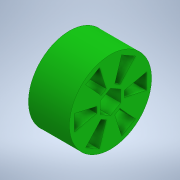
# Autodesk Inventor part: Compliance wheel
Saved by Autodesk Inventor 2021.1 (Build 251245000, 245)
## iProperties
Created: 2020-01-14
Part Number: Compliance wheel
Material: ABS Plastic
Document SubType Name: Modeling
Designer: woodn
Density: 1.06 g/cm^3
Appearance: Dark Green
Author: woodn
Autodesk Inventor part; units mm, degrees
ref_plane "YZ Plane" through (0, 0, 0) normal (1, 0, 0) x (0, 1, 0)
ref_plane "XZ Plane" through (0, 0, 0) normal (0, 1, 0) x (-1, 0, 0)
ref_plane "XY Plane" through (0, 0, 0) normal (0, 0, 1) x (1, 0, 0)
sketch "Sketch1" plane through (0, 0, 0) normal (1, 0, 0) x (0, 1, 0)
  circle A0 centre (0, 0) radius 25.4
  dimension "d16" = 50.8
  constraints: 1 centre point, 1 coincident
  measures "d16" diameter of A0
extrude "Extrusion1" add sketch "Sketch1" along normal blind 25.4
sketch "Sketch2" plane through (25.4, 0, 0) normal (1, 0, 0) x (0, 0, -1)
  circle A0 centre (0, 0) radius 50.8
  circle A1 centre (0, 0) radius 25.4
  line L0 (6.35, 3.6662) -> (6.35, -3.6662)
  line L1 (6.35, -3.6662) -> (0, -7.3323)
  line L2 (0, -7.3323) -> (-6.35, -3.6662)
  line L3 (-6.35, -3.6662) -> (-6.35, 3.6662)
  line L4 (-6.35, 3.6662) -> (0, 7.3323)
  line L5 (0, 7.3323) -> (6.35, 3.6662)
  circle A2 centre (0, 0) radius 44.45
  line L6 (0, 0) -> (-5.6587, 24.7616)
  circle A3 centre (0, 0) radius 25.4 projected
  line L7 (0, 0) -> (5.2266, 24.8564)
  arc A4 (9.1466, 43.4988) -> (-9.9027, 43.3329) centre (0, 0) ccw
  point P0 (5.2266, 24.8564)
  point P1 (-5.6587, 24.7616)
  dimension "d3" = 25.4
  dimension "d4" = 6.35
  dimension "d5" = 0
  dimension "d8" = 6.35
  dimension "d9" = 19.05
  dimension "d10" = 0
  constraints: 16 end point, 6 point on circle, 4 centre point, 2 coincident, 2 point on line, 14 other
  measures "d3" radial gap between concentric circles of A0 A1
  measures "d4" distance from line of point (0, 0) L5
  measures "d5" horizontal distance of point (0, 0) L4.end
  measures "d8" radial gap between concentric circles of A0 A2
  measures "d9" distance of A2.start A2.end
  measures "d10" distance of point (0, 0) A4.centre
extrude "Extrusion4" cut sketch "Sketch2" against normal through all contours L7 L6 L4 L5 | L5 L0 L1 L2 L3 L4 L6 L7
sketch "Sketch3" plane through (25.4, 0, 0) normal (1, 0, 0) x (0, 0, -1)
  line L0 (0, 0) -> (-24.7979, -5.4976)
  circle A0 centre (0, 0) radius 25.4 projected
  line L1 (0, 0) -> (-31.7928, 7.0483)
  line L2 (0, 0) -> (-24.7979, -5.4976)
  line L3 (0, 0) -> (-24.7979, 5.4976)
  line L4 (-22.3038, -4.9446) -> (-22.3038, 4.9446)
  line L5 (-8.5331, -1.8918) -> (-8.5331, 1.8918)
  point P0 (-8.5331, 1.8918)
  point P1 (-22.3038, 4.9446)
  dimension "d19" = 25
  constraints: 12 end point, 5 point on line, 2 point on circle, 1 equal length, 1 parallel, 1 vertical
  measures "d19" angle of L1 L0
extrude "Extrusion5" cut sketch "Sketch3" against normal through all contours L0 L4 L1 L5
pattern_circular "Circular Pattern2" count 6 over 360 about axis through (0, 0, 0) along (1, 0, 0) of "Extrusion5"
body "Solid1"
